Autodesk Inventor part; units mm, degrees
(part 2 of 2)
  dimension "d31" = 1
  dimension "d32" = 11
  constraints: 188 end point, 94 point on circle, 46 centre point, 14 tangent, 6 point on line, 4 horizontal, 3 equal radius, 3 parallel, 2 perpendicular, 2 vertical, 1 coincident, 1 collinear, 122 other
  measures "d16" distance between parallel lines of L208 L240
  measures "d17" diameter of A80
  measures "d20" angle of L328 L329
  measures "d21" distance between parallel lines of L327 L328
  measures "d22" distance between parallel lines of L321 L320
  measures "d23" distance of L321.start point (3.078, 12.115)
  measures "d24" distance of L328.start point (3.078, -12.115)
  measures "d25" distance between parallel lines of L329 L331
  measures "d26" distance of point (3.078, -12.115) point (4.917, -15.667)
  measures "d27" radius of A81
  measures "d28" radius of A84
  measures "d29" distance between parallel lines of L325 L323
  measures "d30" distance between parallel lines of L326 L324
  measures "d31" vertical distance of L324.end A84.centre
  measures "d32" distance from line of L324 A80.centre
extrude "Extrusion4" add sketch "Sketch2" along normal blind 10 contours L327 A59 L278 L277 A58 L276 L275 A57 L274 L273 A56 L272 L271 A55 L270 L269 A54 L268 L267 A53 L266 L265 A52 L264 L263 A51 L262 L261 A50 L260 L259 A49 L258 L257 A48 L320 A80 | A80 L328 A83 L329 A84 A85 L331 A82 L327 | L320 L322 L333 L325 L326 L332 L324 L323 A81 L321 A80
mirror "Mirror1" about plane through (0, 0, 13.1152) normal (1, 0, 0) of "Extrusion4"
sketch "Sketch3" plane through (0, 0, 0) normal (0, -1, 0) x (1, 0, 0)
  line L0 (12, 13.1152) -> (-12, 13.1152) projected
  line L1 (-12, 13.1152) -> (-12, -16.239) projected
  line L2 (-12, -16.239) -> (-11, -16.239) projected
  line L3 (-11, -16.239) -> (-11, 12.1152) projected
  line L4 (11, -16.239) -> (11, 12.1152) projected
  line L5 (12, -16.239) -> (11, -16.239) projected
  line L6 (12, 13.1152) -> (12, -16.239) projected
  line L7 (11, 12.1152) -> (6.0774, 12.1152) projected
  line L8 (-11, 12.1152) -> (11, 12.1152)
  constraints: 2 end point, 1 collinear
extrude "Extrusion5" add sketch "Sketch3" along normal blind 3
sketch "Sketch4" plane through (0, -3, 0) normal (0, -1, 0) x (1, 0, 0)
  line L0 (9.917, -16.239) -> (12, -16.239) projected
  line L1 (12, -16.239) -> (-12, -16.239)
  line L2 (-12, -16.239) -> (-12, 13.1152)
  line L3 (-12, 13.1152) -> (12, 13.1152)
  line L4 (12, 13.1152) -> (12, -16.239)
  point P0 (0, 0)
  point P1 (10.917, -18.239)
  constraints: 8 end point, 2 parallel, 1 horizontal, 1 perpendicular, 1 other
extrude "Extrusion6" add sketch "Sketch4" along normal blind 1
sketch "Sketch5" plane through (0, 10, 0) normal (0, 1, 0) x (1, 0, 0)
  circle A0 centre (0, 0) radius 3.829 construction
  constraints: 1 centre point, 1 coincident
equation "\"try\" = 2.236068"
body "Solid2"
